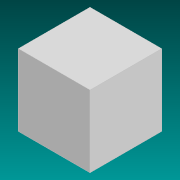
# Autodesk Inventor part: testSven
Saved by Autodesk Inventor 2020.2 (Build 242310000, 310)
## iProperties
Created: 2020-05-15
Part Number: testSven
Material: Generic
Document SubType Name: Modeling
Designer: Svend
Density: 1 g/cm^3
Appearance: Default
Author: Svend
Autodesk Inventor part; units mm, degrees
ref_plane "YZ Plane" through (0, 0, 0) normal (1, 0, 0) x (0, 1, 0)
ref_plane "XZ Plane" through (0, 0, 0) normal (0, 1, 0) x (-1, 0, 0)
ref_plane "XY Plane" through (0, 0, 0) normal (0, 0, 1) x (1, 0, 0)
sketch "Sketch1" plane through (0, 0, 0) normal (0, 0, 1) x (1, 0, 0)
  line L0 (-3, 3) -> (3, 3)
  line L1 (3, 3) -> (3, -3)
  line L2 (3, -3) -> (-3, -3)
  line L3 (-3, -3) -> (-3, 3)
  point P0 (0, 0)
  constraints: 8 end point, 2 parallel, 1 horizontal, 1 perpendicular
extrude "Extrusion1" add sketch "Sketch1" along normal blind 6
body "Solid1"
